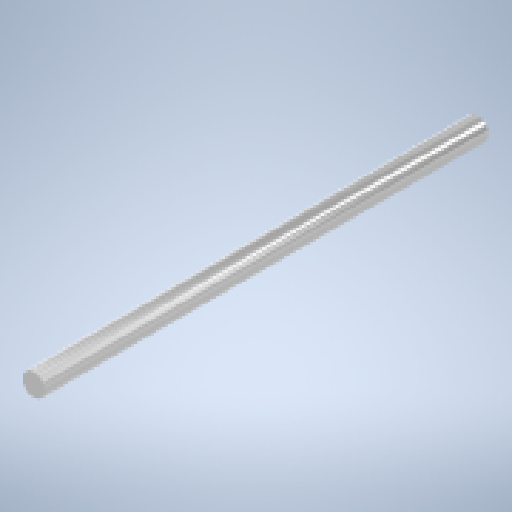
# Autodesk Inventor part: Plate Support
Saved by Autodesk Inventor 2025.3 (Build 293356000, 356)
## iProperties
Created: 2025-10-11
Part Number: Plate Support
Material: Aluminum 6061
Document SubType Name: Modeling
Designer: Haggag
Density: 2.7 g/cm^3
Appearance: Aluminum - Flat
Author: Haggag
Autodesk Inventor part; units mm, degrees
ref_plane "YZ Plane" through (0, 0, 0) normal (1, 0, 0) x (0, 1, 0)
ref_plane "XZ Plane" through (0, 0, 0) normal (0, 1, 0) x (-1, 0, 0)
ref_plane "XY Plane" through (0, 0, 0) normal (0, 0, 1) x (1, 0, 0)
sketch "Sketch1" plane through (0, 0, 0) normal (0, 0, 1) x (1, 0, 0)
  circle A0 centre (0, 0) radius 5.95
  dimension "d1" = 11.9
  constraints: 1 centre point
  measures "d1" diameter of A0
extrude "Extrusion1" add sketch "Sketch1" along normal mid plane 236.69
chamfer "Chamfer3" distance 0.5 angle 45 1 edges at (-5.95, 0, -118.345)
sketch "Sketch4" plane through (0, 0, 118.345) normal (0, 0, 1) x (1, 0, 0)
  circle A0 centre (0, 0) radius 6
  constraints: 1 centre point, 1 coincident
extrude "Extrusion5" add sketch "Sketch4" along normal blind 3
body "Solid1"
